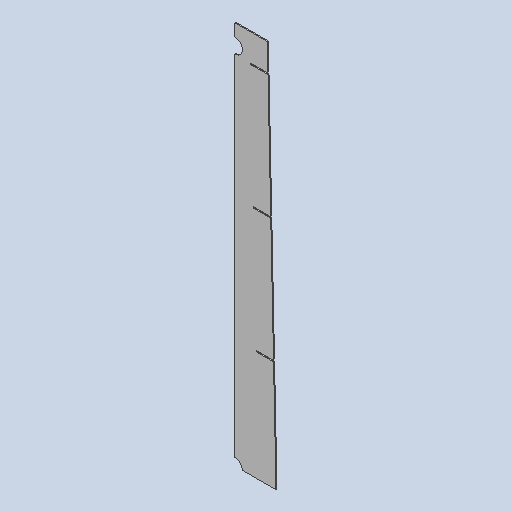
# Autodesk Inventor part: GBK 3201 Center second rib
Saved by Autodesk Inventor 2026.2 (Build 302298000, 298)
## iProperties
Created: 2026-04-17
Part Number: GBK 3201 Center second rib
Material: Steel
Document SubType Name: Sheet Metal
Designer: pokla
Mass: 7201.32 g
Surface Area: 4740.76 cm^2
Volume: 917.366 cm^3
Density: 7.85 g/cm^3
Sheet Metal Rule: Default
Appearance: Default
Flat Pattern Width: 16.6667 cm
Flat Pattern Length: 155.962 cm
Flat Pattern Area: 2599.37 cm^2
Sheet Metal Width: 166,667 mm
Sheet Metal Length: 1559,625 mm
Sheet Metal Area: 259937,430 mm^2
Author: admin
Autodesk Inventor part; units mm, degrees
ref_plane "YZ Plane" through (0, 0, 0) normal (1, 0, 0) x (0, 1, 0)
ref_plane "XZ Plane" through (0, 0, 0) normal (0, 1, 0) x (-1, 0, 0)
ref_plane "XY Plane" through (0, 0, 0) normal (0, 0, 1) x (1, 0, 0)
sketch "Sketch1" plane through (0, 0, 0) normal (0, 0, 1) x (1, 0, 0)
  line L0 (0, 0) -> (0, 4438.8737)
  line L1 (0, 4438.8737) -> (100, 4438.8737)
  line L2 (100, 4438.8737) -> (200, 0)
  line L3 (200, 0) -> (0, 0)
  circle A0 centre (0, 0) radius 30
  line L4 (0, 1479.6246) -> (166.6667, 1479.6246)
  line L5 (0, 2959.2492) -> (133.3333, 2959.2492)
  circle A1 centre (0, 1479.6246) radius 30
  circle A2 centre (0, 2959.2492) radius 30
  line L6 (190.4255, 425) -> (120.4255, 425)
  line L7 (120.4255, 425) -> (120.4255, 430)
  line L8 (120.4255, 430) -> (190.4255, 430)
  line L9 (190.4255, 430) -> (190.4255, 425)
  line L10 (109.1642, 929.8732) -> (179.1642, 929.8732)
  line L11 (179.1642, 924.8732) -> (109.1642, 924.8732)
  line L12 (109.1642, 924.8732) -> (109.1642, 929.8732)
  line L13 (179.1642, 929.8732) -> (179.1642, 924.8732)
  line L14 (97.903, 1429.7463) -> (167.903, 1429.7463)
  line L15 (167.903, 1424.7463) -> (97.903, 1424.7463)
  line L16 (97.903, 1424.7463) -> (97.903, 1429.7463)
  line L17 (167.903, 1429.7463) -> (167.903, 1424.7463)
  line L18 (86.6417, 1929.6195) -> (156.6417, 1929.6195)
  line L19 (156.6417, 1924.6195) -> (86.6417, 1924.6195)
  line L20 (86.6417, 1924.6195) -> (86.6417, 1929.6195)
  line L21 (156.6417, 1929.6195) -> (156.6417, 1924.6195)
  line L22 (75.3805, 2429.4927) -> (145.3805, 2429.4927)
  line L23 (145.3805, 2424.4927) -> (75.3805, 2424.4927)
  line L24 (75.3805, 2424.4927) -> (75.3805, 2429.4927)
  line L25 (145.3805, 2429.4927) -> (145.3805, 2424.4927)
  line L26 (64.1192, 2929.3658) -> (134.1192, 2929.3658)
  line L27 (134.1192, 2924.3658) -> (64.1192, 2924.3658)
  line L28 (64.1192, 2924.3658) -> (64.1192, 2929.3658)
  line L29 (134.1192, 2929.3658) -> (134.1192, 2924.3658)
  line L30 (52.8579, 3429.239) -> (122.8579, 3429.239)
  line L31 (122.8579, 3424.239) -> (52.8579, 3424.239)
  line L32 (52.8579, 3424.239) -> (52.8579, 3429.239)
  line L33 (122.8579, 3429.239) -> (122.8579, 3424.239)
  line L34 (41.5967, 3929.1122) -> (111.5967, 3929.1122)
  line L35 (111.5967, 3924.1122) -> (41.5967, 3924.1122)
  line L36 (41.5967, 3924.1122) -> (41.5967, 3929.1122)
  line L37 (111.5967, 3929.1122) -> (111.5967, 3924.1122)
  line L38 (0, 1629.6246) -> (163.2874, 1629.6246)
  line L39 (0, 3039.2492) -> (131.5311, 3039.2492)
  point P0 (30, 2959.2492)
  point P1 (0, 2929.2492)
  point P2 (0, 1509.6246)
  point P3 (0, 1449.6246)
  point P4 (0, 30)
  point P5 (30, 0)
  point P6 (190.3129, 430)
  point P7 (179.0516, 929.8732)
  point P8 (167.7903, 1429.7463)
  point P9 (30, 1479.6246)
  point P10 (156.5291, 1929.6195)
  point P11 (145.2678, 2429.4927)
  point P12 (134.0066, 2929.3658)
  point P13 (0, 2989.2492)
  dimension "d65" = 100
  dimension "d67" = 200
  dimension "d68" = 60
  dimension "d69" = 1480
  dimension "d70" = 1480
  dimension "d71" = 1480
  dimension "d72" = 5
  dimension "d73" = 70
  dimension "d74" = 430
  dimension "d77" = 500
  dimension "d82" = 80
  dimension "d83" = 150
  measures "d65" distance of L0.end L1.end
  measures "d67" distance of L2.end L0.start
  measures "d68" diameter of A0
  measures "d69" distance of L4.end L2.end
  measures "d70" distance of L4.end L5.end
  measures "d71" distance of L1.end L5.end
  measures "d72" distance of L6.end L7.end
  measures "d73" distance of L6.start L6.end
  measures "d74" distance between parallel lines of L3 L8
  measures "d77" distance of L7.end L10.start
  measures "d82" distance between parallel lines of L5 L39
  measures "d83" distance between parallel lines of L38 L4
extrude "Plate3" add sketch "Sketch1" along normal blind 4 contours L39 L2 L5 A2 L0 | L5 L2 L26 L28 L27 L22 L24 L23 L18 L20 L19 L38 L0 A2 | L38 L2 L4 A1 L0
chamfer "Corner Chamfer2" distance 3 angle 45 6 edges at (156.6417, 1924.6195, 2) (156.5291, 1929.6195, 2) (145.3805, 2424.4927, 2) (145.2678, 2429.4927, 2) (134.1192, 2924.3658, 2) (134.0066, 2929.3658, 2)
equation "\"BendRadius\" = Thickness"
equation "\"BendReliefWidth\" = Thickness"
equation "\"BendReliefDepth\" = 0.5 * Thickness"
equation "\"CornerReliefSize\" = 4 * Thickness"
equation "\"MinimumRemnant\" = 2 * Thickness"
equation "\"TransitionRadius\" = BendRadius"
equation "\"JacobiRadiusSize\" = BendRadius"
equation "\"GapSize\" = Thickness"
equation "\"Thickness\" = 4"
body "Solid2"
